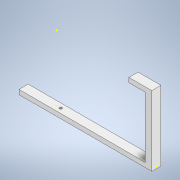
# Autodesk Inventor part: handle
Saved by Autodesk Inventor 2022 (Build 260153070, 153G)
## iProperties
Created: 2021-07-03
Part Number: handle
Material: PBT Plastic
Document SubType Name: Modeling
Designer: AKASH ARYAN
Density: 1.31 g/cm^3
Appearance: Smooth - White
Author: AKASH ARYAN
Autodesk Inventor part; units mm, degrees
ref_plane "YZ Plane" through (0, 0, 0) normal (1, 0, 0) x (0, 1, 0)
ref_plane "XZ Plane" through (0, 0, 0) normal (0, 1, 0) x (-1, 0, 0)
ref_plane "XY Plane" through (0, 0, 0) normal (0, 0, 1) x (1, 0, 0)
sketch "Sketch1" plane through (0, 0, 0) normal (1, 0, 0) x (0, 1, 0)
  line L0 (3.5, -7) -> (-3.5, -7)
  line L1 (-3.5, -7) -> (-3.5, 7)
  line L2 (-3.5, 7) -> (3.5, 7)
  line L3 (3.5, 7) -> (3.5, -7)
  line L4 (3.5, -7) -> (-3.5, 7) construction
  line L5 (-3.5, -7) -> (3.5, 7) construction
  point P0 (0, 0)
  dimension "d0" = 7
  dimension "d1" = 14
  constraints: 12 end point, 2 midpoint, 2 parallel, 1 horizontal, 1 perpendicular
  measures "d0" distance of L1.end L2.end
  measures "d1" distance of L0.end L1.end
extrude "Extrusion1" add sketch "Sketch1" along normal blind 152.4 and the other way blind 50.8
sketch "Sketch2" plane through (-50.8, 3.5, 7) normal (0, 1, 0) x (1, 0, 0)
  circle A0 centre (56.8, 7) radius 2
  point P0 (50.8, 7)
  dimension "d4" = 4
  dimension "d5" = 6
  constraints: 1 centre point
  measures "d4" diameter of A0
  measures "d5" distance of point (50.8, 7) A0.centre
extrude "Extrusion2" cut sketch "Sketch2" against normal through all
sketch "Sketch3" plane through (-50.8, 3.5, 7) normal (0, 1, 0) x (1, 0, 0)
  line L0 (203.2, 0) -> (193.2, 0)
  line L1 (193.2, 0) -> (193.2, 14)
  line L2 (193.2, 14) -> (203.2, 14)
  line L3 (203.2, 14) -> (203.2, 0)
  line L4 (203.2, 0) -> (0, 0) projected
  line L5 (203.2, 14) -> (203.2, 0) projected
  point P0 (50.8, 7)
  dimension "d8" = 10
  dimension "d9" = 14
  dimension "d10" = 0
  dimension "d11" = 0
  constraints: 8 end point, 2 parallel, 1 horizontal, 1 perpendicular
  measures "d8" distance of L1.end L2.end
  measures "d9" distance of L0.end L1.end
  measures "d10" distance between parallel lines of L4 L0
  measures "d11" distance between parallel lines of L5 L3
extrude "Extrusion3" add sketch "Sketch3" along normal blind 100
sketch "Sketch5" plane through (142.4, 3.5, -7) normal (-1, 0, 0) x (0, 0, 1)
  line L0 (14, 100) -> (0, 100)
  line L1 (0, 100) -> (0, 93)
  line L2 (0, 93) -> (14, 93)
  line L3 (14, 93) -> (14, 100)
  line L4 (14, 0) -> (14, 100) projected
  line L5 (0, 100) -> (14, 100) projected
  point P0 (7, -3.5)
  dimension "d17" = 14
  dimension "d18" = 7
  dimension "d19" = 0
  dimension "d20" = 0
  constraints: 8 end point, 2 parallel, 1 horizontal, 1 perpendicular
  measures "d17" distance of L2.end L1.end
  measures "d18" distance of L1.end L0.end
  measures "d19" distance between parallel lines of L4 L3
  measures "d20" distance between parallel lines of L5 L0
extrude "Extrusion4" add sketch "Sketch5" along normal blind 25
sketch "Sketch10" plane through (-50.8, 3.5, 7) normal (0, 1, 0) x (1, 0, 0)
  point P0 (50.8, 7)
sketch "Sketch11" plane through (-50.8, 0, 0) normal (-1, 0, 0) x (0, 0, 1)
  point P0 (0, 0)
sketch "Sketch12" plane through (152.4, 0, 0) normal (1, 0, 0) x (0, 0, -1)
  point P0 (0, 0)
sketch "Sketch13" plane through (-50.8, 103.5, 7) normal (0, 1, 0) x (1, 0, 0)
  point P0 (50.8, 7)
body "Solid1"
